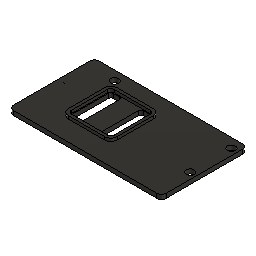
Encoder Mount (Autodesk Fusion 360 design; units mm, degrees)
Autodesk Fusion 360 part; units mm, degrees
note: some values were not read from the file. Set by a fixed rule: which sketch regions a step uses.
sketch "Sketch1" plane through (0, 0, 0) normal (0, 0, 1) x (1, 0, 0)
  circle A0 centre (18.7728, 42.4051) radius 2.159
  line L0 (-60.9197, 30.0451) -> (-60.9197, 58.9153)
  line L1 (22.2603, 30.0451) -> (22.2603, 58.9153)
  circle A1 centre (-44.7272, 19.9053) radius 2.159
  circle A2 centre (18.7728, 19.9051) radius 2.159
  line L2 (-60.9197, 30.0451) -> (-60.9197, 17.3451)
  line L3 (22.2603, 30.0451) -> (22.2603, 17.3451)
  line L4 (19.7203, 14.8051) -> (3.2103, 14.8051)
  line L5 (-41.8697, 14.8051) -> (-58.3797, 14.8051)
  arc A3 (-60.9197, 17.3451) -> (-58.3797, 14.8051) centre (-58.3797, 17.3451) ccw
  arc A4 (19.7203, 14.8051) -> (22.2603, 17.3451) centre (19.7203, 17.3451) ccw
  line L6 (-41.8697, 14.8051) -> (3.2103, 14.8051)
  line L7 (-57.4272, 61.4553) -> (19.7203, 61.4553)
  line L8 (-57.4272, 61.4553) -> (-58.3797, 61.4553)
  arc A5 (-58.3797, 61.4553) -> (-60.9197, 58.9153) centre (-58.3797, 58.9153) ccw
  arc A6 (22.2603, 58.9153) -> (19.7203, 61.4553) centre (19.7203, 58.9153) ccw
  line L9 (-23.0468, 48.4378) -> (-19.6337, 48.4378)
  line L10 (-18.3637, 47.1678) -> (-18.3637, 27.4828)
  line L11 (-40.5887, 27.4828) -> (-40.5887, 47.1678)
  line L12 (-39.3187, 48.4378) -> (-35.9056, 48.4378)
  line L13 (-57.7726, 34.7366) -> (-57.0819, 34.7366)
  line L14 (-34.6356, 38.3051) -> (-34.6356, 47.1678)
  line L15 (-34.6356, 38.3051) -> (-34.6356, 27.4828)
  line L16 (-24.3168, 38.3051) -> (-24.3168, 47.1678)
  line L17 (-24.3168, 38.3051) -> (-24.3168, 27.4828)
  line L18 (-19.6337, 26.2128) -> (-23.0468, 26.2128)
  line L19 (-35.9056, 26.2128) -> (-39.3187, 26.2128)
  arc A7 (-39.3187, 48.4378) -> (-40.5887, 47.1678) centre (-39.3187, 47.1678) ccw
  arc A8 (-34.6356, 47.1678) -> (-35.9056, 48.4378) centre (-35.9056, 47.1678) ccw
  arc A9 (-23.0468, 48.4378) -> (-24.3168, 47.1678) centre (-23.0468, 47.1678) ccw
  arc A10 (-18.3637, 47.1678) -> (-19.6337, 48.4378) centre (-19.6337, 47.1678) ccw
  arc A11 (-19.6337, 26.2128) -> (-18.3637, 27.4828) centre (-19.6337, 27.4828) ccw
  arc A12 (-24.3168, 27.4828) -> (-23.0468, 26.2128) centre (-23.0468, 27.4828) ccw
  arc A13 (-35.9056, 26.2128) -> (-34.6356, 27.4828) centre (-35.9056, 27.4828) ccw
  arc A14 (-40.5887, 27.4828) -> (-39.3187, 26.2128) centre (-39.3187, 27.4828) ccw
  line L20 (-40.5887, 37.3253) -> (-60.9087, 37.3253)
  line L21 (-37.6121, 48.4378) -> (-37.6121, 61.4553)
  arc A15 (-57.0819, 34.7366) -> (-57.7726, 34.7366) centre (-57.4272, 32.6053) ccw
  point P0 (-54.3297, 57.5051)
  point P1 (-60.9197, 27.5051)
  point P2 (-60.9197, 71.9551)
  point P3 (22.2603, 27.5051)
  point P4 (22.2603, 71.9551)
  point P5 (-60.9197, 14.8051)
  point P6 (22.2603, 14.8051)
  point P7 (-18.3637, 48.4378)
  point P8 (-18.3637, 26.2128)
  point P9 (-40.5887, 26.2128)
  point P10 (-40.5887, 48.4378)
  dimension "d37" = 4.318
  dimension "d42" = 4.318
  dimension "d49" = 44.45
  dimension "d51" = 44.45
  dimension "d84" = 4.318
  dimension "d86" = 4.318
  dimension "d89" = 15.24
  dimension "d90" = 15.24
  dimension "d93" = 2.54
  dimension "d139" = 2.54
  dimension "d142" = 22.225
  dimension "d143" = 22.225
  dimension "d144" = 22.225
  dimension "d146" = 10.3188
  dimension "d149" = 1.27
  dimension "d155" = 20.32
  dimension "d156" = 13.0175
  constraint coincident P2 L0
  constraint coincident P4 L1
  constraint coincident P3 L1
  constraint coincident P1 L0
  constraint collinear L4 L5
  constraint coincident P5 L2
  constraint coincident P5 L5
  constraint tangent L2 A3
  constraint tangent L5 A3
  constraint coincident P6 L3
  constraint coincident P6 L4
  constraint tangent L3 A4
  constraint tangent L4 A4
  constraint equal A3 A4
  constraint perpendicular L0 L13
  constraint perpendicular L1 L7
  constraint perpendicular L0 L8
  constraint tangent L8 A5
  constraint tangent L0 A5
  constraint tangent L7 A6
  constraint tangent L1 A6
  constraint equal A5 A6
  constraint perpendicular L9 L10
  constraint perpendicular L10 L18
  constraint perpendicular L11 L18
  constraint perpendicular L7 L14
  constraint perpendicular L6 L15
  constraint perpendicular L7 L16
  constraint perpendicular L6 L17
  constraint collinear L18 L19
  constraint coincident P10 L11
  constraint coincident P10 L12
  constraint tangent L11 A7
  constraint tangent L12 A7
  constraint tangent L14 A8
  constraint tangent L12 A8
  constraint equal A7 A8
  constraint tangent L16 A9
  constraint tangent L9 A9
  constraint equal A7 A9
  constraint coincident P7 L9
  constraint coincident P7 L10
  constraint tangent L9 A10
  constraint tangent L10 A10
  constraint equal A7 A10
  constraint coincident P8 L10
  constraint coincident P8 L18
  constraint tangent L10 A11
  constraint tangent L18 A11
  constraint equal A7 A11
  constraint tangent L18 A12
  constraint tangent L17 A12
  constraint equal A7 A12
  constraint tangent L19 A13
  constraint tangent L15 A13
  constraint equal A7 A13
  constraint coincident P9 L19
  constraint coincident P9 L11
  constraint tangent L19 A14
  constraint tangent L11 A14
  constraint equal A7 A14
  constraint midpoint L11 L20.start
  constraint perpendicular L0 L20
  constraint midpoint L12 L21.start
  constraint perpendicular L7 L21
  constraint coincident L7 L21.end
  measures "d37" diameter of A0
  measures "d42" diameter of A15
  measures "d49" distance of P1 P2
  measures "d51" distance of P3 P4
  measures "d84" diameter of A1
  measures "d86" diameter of A2
  measures "d89" distance of L0.start P5
  measures "d90" distance of L1.start P6
  measures "d93" radius of A3
  measures "d139" radius of A5
  measures "d142" distance of P7 P8
  measures "d143" distance of P8 P9
  measures "d144" distance of P9 P10
  measures "d146" distance of L16.start L14.start
  measures "d149" radius of A7
  measures "d155" distance of L20.start L20.end
  measures "d156" distance of L21.start L21.end
extrude "Extrude11" add sketch "Sketch1" along normal blind 2.3813
sketch "Sketch10" plane through (0, 0, 2.3813) normal (0, 0, 1) x (-1, 0, 0)
  circle A0 centre (44.7272, -19.9053) radius 2.159
  circle A1 centre (-18.7728, -19.9051) radius 2.159
  circle A2 centre (-18.7728, -42.4051) radius 2.159
  line L0 (24.3168, -27.4828) -> (24.3168, -47.1678)
  line L1 (23.0468, -48.4378) -> (19.6337, -48.4378)
  line L2 (18.3637, -47.1678) -> (18.3637, -27.4828)
  line L3 (35.9056, -26.2128) -> (39.3187, -26.2128)
  line L4 (34.6356, -47.1678) -> (34.6356, -27.4828)
  line L5 (40.5887, -27.4828) -> (40.5887, -47.1678)
  line L6 (39.3187, -48.4378) -> (35.9056, -48.4378)
  line L7 (-22.2603, -17.3451) -> (-22.2603, -58.9153)
  arc A3 (-22.2603, -58.9153) -> (-19.7203, -61.4553) centre (-19.7203, -58.9153) ccw
  line L8 (-19.7203, -61.4553) -> (58.3797, -61.4553)
  arc A4 (58.3797, -61.4553) -> (60.9197, -58.9153) centre (58.3797, -58.9153) ccw
  line L9 (60.9197, -58.9153) -> (60.9197, -17.3451)
  arc A5 (60.9197, -17.3451) -> (58.3797, -14.8051) centre (58.3797, -17.3451) ccw
  line L10 (58.3797, -14.8051) -> (-19.7203, -14.8051)
  arc A6 (-19.7203, -14.8051) -> (-22.2603, -17.3451) centre (-19.7203, -17.3451) ccw
  arc A7 (39.3187, -48.4378) -> (40.5887, -47.1678) centre (39.3187, -47.1678) ccw
  arc A8 (34.6356, -47.1678) -> (35.9056, -48.4378) centre (35.9056, -47.1678) ccw
  arc A9 (35.9056, -26.2128) -> (34.6356, -27.4828) centre (35.9056, -27.4828) ccw
  arc A10 (40.5887, -27.4828) -> (39.3187, -26.2128) centre (39.3187, -27.4828) ccw
  arc A11 (23.0468, -48.4378) -> (24.3168, -47.1678) centre (23.0468, -47.1678) ccw
  arc A12 (18.3637, -47.1678) -> (19.6337, -48.4378) centre (19.6337, -47.1678) ccw
  arc A13 (19.6337, -26.2128) -> (18.3637, -27.4828) centre (19.6337, -27.4828) ccw
  line L11 (19.6337, -26.2128) -> (23.0468, -26.2128)
  arc A14 (24.3168, -27.4828) -> (23.0468, -26.2128) centre (23.0468, -27.4828) ccw
  line L12 (39.3264, -48.4391) -> (19.6414, -48.4391)
  line L13 (18.3714, -47.1691) -> (18.3714, -27.4841)
  line L14 (19.6414, -26.2141) -> (39.3264, -26.2141)
  line L15 (40.5964, -27.4841) -> (40.5964, -47.1691)
  arc A15 (39.3264, -48.4391) -> (40.5964, -47.1691) centre (39.3264, -47.1691) ccw
  arc A16 (18.3714, -47.1691) -> (19.6414, -48.4391) centre (19.6414, -47.1691) ccw
  arc A17 (19.6414, -26.2141) -> (18.3714, -27.4841) centre (19.6414, -27.4841) ccw
  arc A18 (40.5964, -27.4841) -> (39.3264, -26.2141) centre (39.3264, -27.4841) ccw
  line L16 (19.6414, -25.6849) -> (39.3264, -25.6849)
  arc A19 (41.1255, -27.4841) -> (39.3264, -25.6849) centre (39.3264, -27.4841) ccw
  line L17 (41.1255, -27.4841) -> (41.1255, -47.1691)
  arc A20 (39.3264, -48.9683) -> (41.1255, -47.1691) centre (39.3264, -47.1691) ccw
  line L18 (39.3264, -48.9683) -> (19.6414, -48.9683)
  arc A21 (17.8422, -47.1691) -> (19.6414, -48.9683) centre (19.6414, -47.1691) ccw
  line L19 (17.8422, -47.1691) -> (17.8422, -27.4841)
  arc A22 (19.6414, -25.6849) -> (17.8422, -27.4841) centre (19.6414, -27.4841) ccw
  arc A23 (16.2547, -47.1691) -> (19.6414, -50.5558) centre (19.6414, -47.1691) ccw
  line L20 (39.3264, -50.5558) -> (19.6414, -50.5558)
  arc A24 (39.3264, -50.5558) -> (42.713, -47.1691) centre (39.3264, -47.1691) ccw
  line L21 (42.713, -27.4841) -> (42.713, -47.1691)
  arc A25 (42.713, -27.4841) -> (39.3264, -24.0974) centre (39.3264, -27.4841) ccw
  line L22 (19.6414, -24.0974) -> (39.3264, -24.0974)
  arc A26 (19.6414, -24.0974) -> (16.2547, -27.4841) centre (19.6414, -27.4841) ccw
  line L23 (16.2547, -47.1691) -> (16.2547, -27.4841)
  arc A27 (57.0819, -34.7366) -> (57.7726, -34.7366) centre (57.4272, -32.6053) ccw
  line L24 (57.0819, -34.7366) -> (57.7726, -34.7366)
  dimension "d150" = -0.5292
  dimension "d151" = 1.27
  dimension "d154" = -1.5875
  constraint perpendicular L2 L12
  constraint perpendicular L11 L13
  constraint perpendicular L5 L14
  constraint perpendicular L12 L15
  constraint tangent L12 A15
  constraint tangent L15 A15
  constraint tangent L12 A16
  constraint tangent L13 A16
  constraint equal A15 A16
  constraint tangent L13 A17
  constraint tangent L14 A17
  constraint equal A15 A17
  constraint tangent L14 A18
  constraint tangent L15 A18
  constraint equal A15 A18
  measures "d151" radius of A15
extrude "Extrude12" add sketch "Sketch10" against normal blind 3.9688 contours A23 L20 A24 L21 A25 L22 A26 L23
move_body "Move1" bodies 1 to x (1, 0, 0) y (0, -1, 0) z (0, 0, -1) at (0, 51.5532, 4.7625)
equation "d142 = ( 7 / 8 ) * 1 in"
equation "d143 = ( 7 / 8 ) * 1 in"
equation "d144 = ( 7 / 8 ) * 1 in"
equation "d146 = ( 13 / 32 ) * 1 in"
equation "d147 = ( 3 / 32 ) * 1 in"
equation "d150 = ( -1 / 48 ) * 1 in"
equation "d152 = ( -5 / 32 ) * 1 in"
equation "d154 = ( -1 / 16 ) * 1 in"
named bodies: "EncoderMount"
